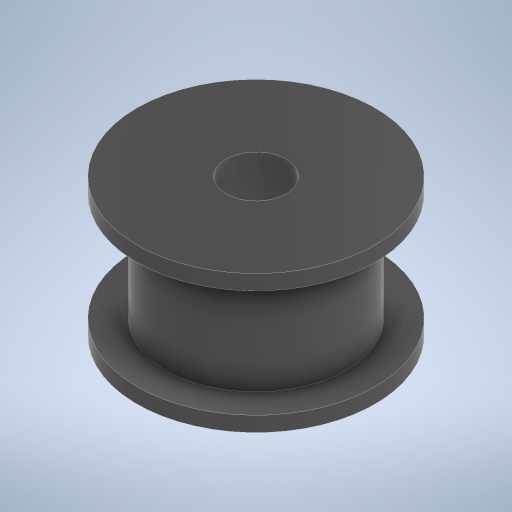
# Autodesk Inventor part: Pulley
Saved by Autodesk Inventor 2023 (Build 270158000, 158)
## iProperties
Created: 2023-03-07
Part Number: Pulley
Material: Типовые
Document SubType Name: Modeling
Designer: Josh
Density: 1 g/cm^3
Appearance: Темно-серый
Author: Josh
Autodesk Inventor part; units mm, degrees
ref_plane "YZ Plane" through (0, 0, 0) normal (1, 0, 0) x (0, 1, 0)
ref_plane "XZ Plane" through (0, 0, 0) normal (0, 1, 0) x (-1, 0, 0)
ref_plane "XY Plane" through (0, 0, 0) normal (0, 0, 1) x (1, 0, 0)
sketch "Эскиз1" plane through (0, 0, 0) normal (0, 1, 0) x (-1, 0, 0)
  circle A0 centre (0, 0) radius 7.9
  circle A1 centre (0, 0) radius 2
  circle A2 centre (0, 0) radius 6
  dimension "d0" = 15.8
  dimension "d1" = 4
  dimension "d4" = 12
  constraints: 3 centre point, 3 coincident
  measures "d0" diameter of A0
  measures "d1" diameter of A1
  measures "d4" diameter of A2
extrude "Выдавливание1" add sketch "Эскиз1" along normal mid plane 9.15 contours A0 | A2
extrude "Выдавливание2" cut sketch "Эскиз1" along normal mid plane 7.15 contours A0
